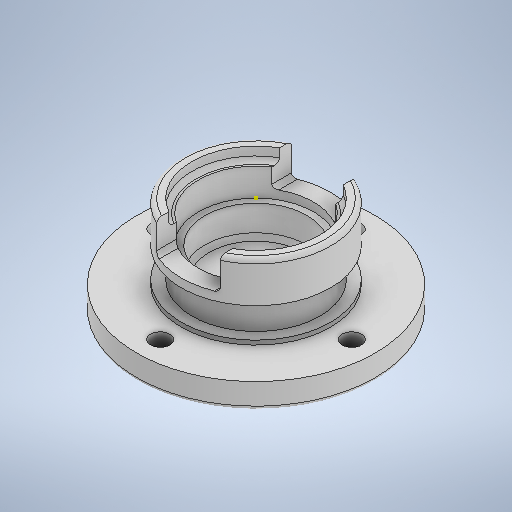
# Autodesk Inventor part: Bai_14
Saved by Autodesk Inventor 2025.1 (Build 291241000, 241)
## iProperties
Created: 2024-10-02
Part Number: Bai_14
Material: Generic
Document SubType Name: Modeling
Designer: msi
Density: 1 g/cm^3
Appearance: Default
Author: msi
Autodesk Inventor part; units mm, degrees
ref_plane "YZ Plane" through (0, 0, 0) normal (1, 0, 0) x (0, 1, 0)
ref_plane "XZ Plane" through (0, 0, 0) normal (0, 1, 0) x (-1, 0, 0)
ref_plane "XY Plane" through (0, 0, 0) normal (0, 0, 1) x (1, 0, 0)
sketch "Sketch1" plane through (0, 0, 0) normal (0, 0, 1) x (1, 0, 0)
  point P0 (0, 0)
sketch "Sketch2" plane through (0, 0, 0) normal (0, 0, 1) x (1, 0, 0)
  line L0 (0, 0) -> (33, 0) construction
  line L1 (35, -2) -> (35, -6)
  line L2 (0, 0) -> (30, 0) construction
  line L3 (0, 0) -> (27, 0) construction
  line L4 (30, 0) -> (30, -4)
  line L5 (35, 0) -> (35, -35) construction
  line L6 (35, -35) -> (35, -47) construction
  line L7 (35, -35) -> (0, -35) construction
  line L8 (0, 0) -> (0, -15) construction
  line L9 (0, 0) -> (15, 0) construction
  line L10 (0, -15) -> (0.4118, -15)
  line L11 (15, 0) -> (15, -13)
  line L12 (0, -15) -> (0.7268, -15)
  line L13 (0.7268, -15) -> (13, -15)
  line L14 (28, -6) -> (15, -6)
  line L15 (35, -35) -> (35, -33)
  line L16 (35, -33) -> (35, -19) construction
  line L17 (35, -19) -> (27, -19)
  line L18 (27, -19) -> (27, -6)
  line L19 (22, -33) -> (0, -33)
  line L20 (35, -19) -> (30, -19)
  line L21 (30, -19) -> (30, -33)
  line L22 (27, -19) -> (24, -19)
  line L23 (24, -19) -> (24, -31)
  line L24 (0, -35) -> (45, -35) construction
  line L25 (45, -35) -> (45, -44) construction
  line L26 (45, -47) -> (0, -47)
  line L27 (45, -47) -> (45, -44) construction
  line L28 (45, -35) -> (56, -35)
  line L29 (56, -35) -> (56, -45)
  line L30 (54, -47) -> (45, -47)
  line L31 (0, -47) -> (0, -44)
  line L32 (0, -44) -> (24, -44) construction
  line L33 (45, -35) -> (49.5, -35)
  line L34 (45, -35) -> (40.5, -35)
  line L35 (40.5, -35) -> (40.5, -44)
  line L36 (49.5, -35) -> (49.5, -44)
  line L37 (0, -47) -> (27, -47)
  line L38 (27, -47) -> (27, -47)
  line L39 (0, -44) -> (27, -44) construction
  line L40 (15, 0) -> (30, 0)
  line L41 (35, 0) -> (30, 0) construction
  line L42 (35, -6) -> (35, -19)
  arc A0 (35, -2) -> (33, 0) centre (33, -2) ccw
  line L43 (30, 0) -> (33, 0)
  arc A1 (28, -6) -> (30, -4) centre (28, -4) ccw
  arc A2 (13, -15) -> (15, -13) centre (13, -13) ccw
  arc A3 (22, -33) -> (24, -31) centre (22, -31) ccw
  line L44 (22, -33) -> (35, -33)
  line L45 (0, -15) -> (0, -47)
  line L46 (35, -44) -> (56, -44) construction
  line L47 (35, -44) -> (35, -47) construction
  arc A4 (54, -47) -> (56, -45) centre (54, -45) ccw
  line L48 (45, -44) -> (54, -44)
  line L49 (54, -44) -> (54, -47)
  line L50 (45, -44) -> (36, -44)
  line L51 (36, -44) -> (36, -47)
  line L52 (27, -47) -> (24, -44)
  line L53 (35, -35) -> (40.5, -35)
  line L54 (0, -44) -> (24, -44)
  line L55 (0, 24.6653) -> (0, -83.972)
  line L56 (0, 0) -> (-15, 0)
  line L57 (-15, 0) -> (-15, -13)
  line L58 (-13, -15) -> (0, -15)
  arc A5 (-15, -13) -> (-13, -15) centre (-13, -13) ccw
  line L59 (15, 0) -> (0, 0)
  point P0 (15, -15)
  point P1 (-15, -6.5)
  dimension "d0" = 35
  dimension "d1" = 6
  dimension "d2" = 30
  dimension "d3" = 27
  dimension "d4" = 35
  dimension "d7" = 15
  dimension "d8" = 15
  dimension "d9" = 2
  dimension "d10" = 14
  dimension "d11" = 8
  dimension "d12" = 5
  dimension "d13" = 3
  dimension "d15" = 3
  dimension "d16" = 11
  dimension "d20" = 27
  dimension "d21" = 2
  dimension "d22" = 2
  dimension "d23" = 2
  dimension "d24" = 2
  dimension "d25" = 2
  dimension "d28" = 3
  dimension "d29" = 3
  dimension "d40" = 2
  constraints: 118 end point, 26 point on line, 18 vertical, 12 horizontal, 12 perpendicular, 12 point on circle, 12 tangent, 7 collinear, 6 centre point, 1 midpoint, 1 parallel, 11 other
  measures "d0" distance of L0.start L5.start
  measures "d1" distance of L5.start L1.end
  measures "d2" distance of L0.start L2.end
  measures "d3" distance of L0.start L3.end
  measures "d4" distance of L5.start L5.end
  measures "d7" distance of L0.start L9.end
  measures "d8" distance of L9.end point (15, -15)
  measures "d9" distance of L5.end L15.end
  measures "d10" distance of L15.end L16.end
  measures "d11" distance of L16.end L17.end
  measures "d12" distance of L16.end L20.end
  measures "d13" distance of L17.end L22.end
  measures "d15" distance of L25.end L26.start
  measures "d16" distance of L24.end L28.end
  measures "d20" distance of L26.end L37.end
  measures "d21" radius of A0
  measures "d22" radius of A1
  measures "d23" radius of A2
  measures "d24" radius of A3
  measures "d25" radius of A4
  measures "d28" distance of L38.end point (27, -44)
  measures "d29" distance of L52.end point (27, -44)
  measures "d40" radius of A5
revolve "Revolution1" add sketch "Sketch2" angle 360 about axis through (0, -15, 0) along (0, -1, 0) contours L1 L42 L17 L18 L14 A1 L4 L43 A0 | L21 L44 A3 L23 L22 L17 | L44 L15 L53 L35 L50 L51 L26 L52 L54 L45 L19 | L34 L28 L36 L48 L50 L35 | L28 L29 A4 L49 L48 L36
sketch "Sketch3" plane through (0, 0, 0) normal (0, 1, 0) x (1, 0, 0)
  circle A0 centre (0, 0) radius 45
  circle A1 centre (0, 45) radius 4.5
  circle A2 centre (-45, 0) radius 4.5
  circle A3 centre (0, -45) radius 4.5
  circle A4 centre (45, 0) radius 4.5
  dimension "d31" = 90
  dimension "d32" = 9
  dimension "d35" = 360
  constraints: 4 centre point, 1 coincident, 1 vertical alignment, 11 other
  measures "d32" diameter of A1
extrude "Extrusion1" cut sketch "Sketch3" against normal blind 49 contours A0 A4 | A0 A4 | A1 A0 | A0 A1 | A3 A0 | A0 A3 | A2 A0 | A0 A2
extrude "Extrusion2" cut sketch "Sketch2" along normal mid plane 112 contours L11 A2 L13 L12 L10 L55 L59 | L55 L58 A5 L57 L56
equation "\"d29\" = d28"
body "Solid1"
